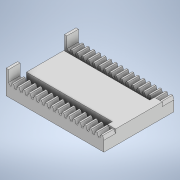
# Autodesk Inventor part: bolt
Saved by Autodesk Inventor 2021 (Build 250183000, 183)
## iProperties
Created: 2024-03-19
Part Number: bolt
Material: Generic
Document SubType Name: Modeling
Designer: 22hamfri
Density: 1 g/cm^3
Appearance: Default
Author: 22hamfri
Autodesk Inventor part; units mm, degrees
ref_plane "YZ Plane" through (0, 0, 0) normal (1, 0, 0) x (0, 1, 0)
ref_plane "XZ Plane" through (0, 0, 0) normal (0, 1, 0) x (-1, 0, 0)
ref_plane "XY Plane" through (0, 0, 0) normal (0, 0, 1) x (1, 0, 0)
sketch "Sketch1" plane through (0, 0, 0) normal (0, 1, 0) x (-1, 0, 0)
  line L0 (-24.5, 11.75) -> (24.5, 11.75)
  line L1 (24.5, 11.75) -> (24.5, -11.75)
  line L2 (24.5, -11.75) -> (-24.5, -11.75)
  line L3 (-24.5, -11.75) -> (-24.5, 11.75)
  line L4 (-24.5, 11.75) -> (24.5, -11.75) construction
  line L5 (24.5, 11.75) -> (-24.5, -11.75) construction
  line L6 (-24.5, -11.75) -> (-29.5, -11.75)
  line L7 (-29.5, -11.75) -> (-29.5, 0)
  line L8 (-29.5, 0) -> (-24.5, 0)
  line L9 (-24.5, 0) -> (-24.5, -11.75)
  line L10 (-29.5, 0) -> (-34.5, 0)
  line L11 (-34.5, 0) -> (-34.5, -22)
  line L12 (-34.5, -22) -> (-29.5, -22)
  line L13 (-29.5, -22) -> (-29.5, 0)
  line L14 (-34.5, 0) -> (24.5, 0)
  line L15 (-29.5, -22) -> (25.5, -22)
  line L16 (25.5, -22) -> (25.5, -14.75)
  line L17 (25.5, -14.75) -> (-29.5, -14.75)
  line L18 (-29.5, -14.75) -> (-29.5, -22)
  line L19 (25.5, -22) -> (27, -22)
  line L20 (27, -22) -> (27, -14.75)
  line L21 (27, -14.75) -> (25.5, -14.75)
  line L22 (25.5, -14.75) -> (25.5, -22)
  line L23 (24.5, 11.75) -> (-24.5, 11.75)
  line L24 (-24.5, 11.75) -> (-29.5, 11.75)
  line L25 (-29.5, 11.75) -> (-29.5, 0)
  line L26 (-24.5, 0) -> (-24.5, 11.75)
  line L27 (-34.5, 0) -> (-34.5, 22)
  line L28 (-34.5, 22) -> (-29.5, 22)
  line L29 (-29.5, 22) -> (-29.5, 0)
  line L30 (-29.5, 22) -> (25.5, 22)
  line L31 (25.5, 22) -> (25.5, 14.75)
  line L32 (25.5, 14.75) -> (-29.5, 14.75)
  line L33 (-29.5, 14.75) -> (-29.5, 22)
  line L34 (25.5, 22) -> (27, 22)
  line L35 (27, 22) -> (27, 14.75)
  line L36 (27, 14.75) -> (25.5, 14.75)
  line L37 (25.5, 14.75) -> (25.5, 22)
  line L38 (-29.5, -14.75) -> (-34.5, -14.75)
  line L39 (-29.5, 14.75) -> (-34.5, 14.75)
  point P0 (0, 0)
  point P1 (-29.5, -14.75)
  dimension "d0" = 49
  dimension "d1" = 23.5
  dimension "d2" = 5
  dimension "d4" = 1.5
  dimension "d5" = 3
  dimension "d7" = 44
  dimension "d29" = 61.5
  dimension "d30" = 5
  constraints: 80 end point, 10 parallel, 9 symmetric about line, 8 perpendicular, 5 horizontal, 3 midpoint, 2 point on line, 1 collinear
  measures "d0" distance between parallel lines of L1 L3
  measures "d1" distance between parallel lines of L2 L0
  measures "d2" distance between parallel lines of L3 L7
  measures "d4" distance between parallel lines of L20 L16
  measures "d5" distance between parallel lines of L17 L2
  measures "d7" distance between parallel lines of L15 L30
  measures "d29" distance between parallel lines of L11 L20
  measures "d30" distance between parallel lines of L11 L13
extrude "Extrusion1" add sketch "Sketch1" along normal blind 9 contours L0 L1 L14 L3 | L3 L8 L25 L24 | L14 L1 L2 L3 | L3 L6 L7 L8 | L25 L10 L27 L39 L29 | L7 L13 L38 L11 L10
extrude "Extrusion2" add sketch "Sketch1" along normal blind 6.5 contours L39 L27 L28 L29 | L29 L30 L31 L32 | L17 L16 L15 L13 | L13 L12 L11 L38
extrude "Extrusion3" add sketch "Sketch1" along normal blind 15 contours L31 L34 L35 L36 | L21 L20 L19 L16
sketch "Sketch2" plane through (34.5, 0, -22) normal (0, 0, -1) x (-1, 0, 0)
  line L0 (0, 6.5) -> (60, 6.5) projected
  line L1 (0, 6.5) -> (0.75, 8.7)
  line L2 (0.75, 8.7) -> (1.25, 8.7)
  line L3 (1.25, 8.7) -> (1.25, 6.5)
  line L4 (1.25, 8.7) -> (1.75, 8.7)
  line L5 (1.75, 8.7) -> (2.5, 6.5)
  line L6 (3.5, 6.5) -> (4.25, 8.7)
  line L7 (4.25, 8.7) -> (4.75, 8.7)
  line L8 (4.75, 8.7) -> (5.25, 8.7)
  line L9 (5.25, 8.7) -> (6, 6.5)
  line L10 (4.75, 8.7) -> (4.75, 6.5)
  line L11 (7, 6.5) -> (7.75, 8.7)
  line L12 (7.75, 8.7) -> (8.25, 8.7)
  line L13 (8.25, 8.7) -> (8.75, 8.7)
  line L14 (8.75, 8.7) -> (9.5, 6.5)
  line L15 (8.25, 8.7) -> (8.25, 6.5)
  line L16 (10.5, 6.5) -> (11.25, 8.7)
  line L17 (11.25, 8.7) -> (11.75, 8.7)
  line L18 (11.75, 8.7) -> (12.25, 8.7)
  line L19 (12.25, 8.7) -> (13, 6.5)
  line L20 (11.75, 8.7) -> (11.75, 6.5)
  line L21 (14, 6.5) -> (14.75, 8.7)
  line L22 (14.75, 8.7) -> (15.25, 8.7)
  line L23 (15.25, 8.7) -> (15.75, 8.7)
  line L24 (15.75, 8.7) -> (16.5, 6.5)
  line L25 (15.25, 8.7) -> (15.25, 6.5)
  line L26 (17.5, 6.5) -> (18.25, 8.7)
  line L27 (18.25, 8.7) -> (18.75, 8.7)
  line L28 (18.75, 8.7) -> (19.25, 8.7)
  line L29 (19.25, 8.7) -> (20, 6.5)
  line L30 (18.75, 8.7) -> (18.75, 6.5)
  line L31 (21, 6.5) -> (21.75, 8.7)
  line L32 (21.75, 8.7) -> (22.25, 8.7)
  line L33 (22.25, 8.7) -> (22.75, 8.7)
  line L34 (22.75, 8.7) -> (23.5, 6.5)
  line L35 (22.25, 8.7) -> (22.25, 6.5)
  line L36 (24.5, 6.5) -> (25.25, 8.7)
  line L37 (25.25, 8.7) -> (25.75, 8.7)
  line L38 (25.75, 8.7) -> (26.25, 8.7)
  line L39 (26.25, 8.7) -> (27, 6.5)
  line L40 (25.75, 8.7) -> (25.75, 6.5)
  line L41 (28, 6.5) -> (28.75, 8.7)
  line L42 (28.75, 8.7) -> (29.25, 8.7)
  line L43 (29.25, 8.7) -> (29.75, 8.7)
  line L44 (29.75, 8.7) -> (30.5, 6.5)
  line L45 (29.25, 8.7) -> (29.25, 6.5)
  line L46 (31.5, 6.5) -> (32.25, 8.7)
  line L47 (32.25, 8.7) -> (32.75, 8.7)
  line L48 (32.75, 8.7) -> (33.25, 8.7)
  line L49 (33.25, 8.7) -> (34, 6.5)
  line L50 (32.75, 8.7) -> (32.75, 6.5)
  line L51 (35, 6.5) -> (35.75, 8.7)
  line L52 (35.75, 8.7) -> (36.25, 8.7)
  line L53 (36.25, 8.7) -> (36.75, 8.7)
  line L54 (36.75, 8.7) -> (37.5, 6.5)
  line L55 (36.25, 8.7) -> (36.25, 6.5)
  line L56 (38.5, 6.5) -> (39.25, 8.7)
  line L57 (39.25, 8.7) -> (39.75, 8.7)
  line L58 (39.75, 8.7) -> (40.25, 8.7)
  line L59 (40.25, 8.7) -> (41, 6.5)
  line L60 (39.75, 8.7) -> (39.75, 6.5)
  line L61 (42, 6.5) -> (42.75, 8.7)
  line L62 (42.75, 8.7) -> (43.25, 8.7)
  line L63 (43.25, 8.7) -> (43.75, 8.7)
  line L64 (43.75, 8.7) -> (44.5, 6.5)
  line L65 (43.25, 8.7) -> (43.25, 6.5)
  line L66 (45.5, 6.5) -> (46.25, 8.7)
  line L67 (46.25, 8.7) -> (46.75, 8.7)
  line L68 (46.75, 8.7) -> (47.25, 8.7)
  line L69 (47.25, 8.7) -> (48, 6.5)
  line L70 (46.75, 8.7) -> (46.75, 6.5)
  line L71 (49, 6.5) -> (49.75, 8.7)
  line L72 (49.75, 8.7) -> (50.25, 8.7)
  line L73 (50.25, 8.7) -> (50.75, 8.7)
  line L74 (50.75, 8.7) -> (51.5, 6.5)
  line L75 (50.25, 8.7) -> (50.25, 6.5)
  line L76 (52.5, 6.5) -> (53.25, 8.7)
  line L77 (53.25, 8.7) -> (53.75, 8.7)
  line L78 (53.75, 8.7) -> (54.25, 8.7)
  line L79 (54.25, 8.7) -> (55, 6.5)
  line L80 (53.75, 8.7) -> (53.75, 6.5)
  line L81 (56, 6.5) -> (56.75, 8.7)
  line L82 (56.75, 8.7) -> (57.25, 8.7)
  line L83 (57.25, 8.7) -> (57.75, 8.7)
  line L84 (57.75, 8.7) -> (58.5, 6.5)
  line L85 (57.25, 8.7) -> (57.25, 6.5)
  point P0 (34.5, 0)
  point P1 (56, 6.5)
  point P2 (58.5, 6.5)
  point P3 (52.5, 6.5)
  point P4 (55, 6.5)
  point P5 (49, 6.5)
  point P6 (51.5, 6.5)
  point P7 (45.5, 6.5)
  point P8 (48, 6.5)
  point P9 (42, 6.5)
  point P10 (44.5, 6.5)
  point P11 (38.5, 6.5)
  point P12 (41, 6.5)
  point P13 (35, 6.5)
  point P14 (37.5, 6.5)
  point P15 (31.5, 6.5)
  point P16 (34, 6.5)
  point P17 (28, 6.5)
  point P18 (30.5, 6.5)
  point P19 (24.5, 6.5)
  point P20 (27, 6.5)
  point P21 (21, 6.5)
  point P22 (23.5, 6.5)
  point P23 (17.5, 6.5)
  point P24 (20, 6.5)
  point P25 (14, 6.5)
  point P26 (16.5, 6.5)
  point P27 (10.5, 6.5)
  point P28 (13, 6.5)
  point P29 (7, 6.5)
  point P30 (9.5, 6.5)
  point P31 (3.5, 6.5)
  point P32 (6, 6.5)
  dimension "d14" = 2.2
  dimension "d15" = 1
  dimension "d18" = 3.5
  dimension "d23" = 2.5
  constraints: 170 end point, 96 horizontal alignment, 48 parallel, 32 collinear, 17 point on line, 1 horizontal, 1 perpendicular, 4 other
  measures "d15" distance of L4.end L1.end
  measures "d18" distance of L1.start L6.start
  measures "d23" distance of L1.start L5.end
extrude "Extrusion4" add sketch "Sketch2" against normal up to surface (7.25 mm away)
mirror "Mirror1" about plane through (0, 0, 0) normal (0, 0, 1) of "Extrusion4"
chamfer "Chamfer1" distance 1.5 angle 45 2 edges at (-25.5, 6.5, -18.375) (-25.5, 6.5, 18.375)
body "Solid1"
